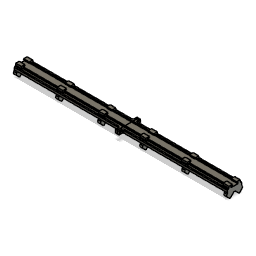
UlTi_LED_Stand (Autodesk Fusion 360 design; units mm, degrees)
Autodesk Fusion 360 part; units mm, degrees
note: some values were not read from the file. Chosen so that the rebuilt part matches the saved one: which bodies a step acts on. Set by a fixed rule: which face or edge a step refers to.
sketch "Sketch1" plane through (0, 0, 0) normal (0, 1, 0) x (1, 0, 0)
  line L0 (0, 0) -> (-300, 0)
  line L1 (-300, 0) -> (-300, 20)
  line L2 (-300, 20) -> (0, 20)
  line L3 (0, 20) -> (0, 0)
  line L4 (-300, 10) -> (0, 10)
  line L5 (-300, 10) -> (-300, 14)
  line L6 (-300, 14) -> (0, 14)
  line L7 (0, 14) -> (0, 6)
  line L8 (0, 6) -> (-300, 6)
  line L9 (-300, 6) -> (-300, 14)
  line L10 (-300, 14) -> (-292, 14)
  line L11 (-292, 14) -> (-292, 18)
  line L12 (-292, 18) -> (-300, 18)
  line L13 (-300, 18) -> (-300, 14)
  line L14 (-300, 16) -> (-292, 16)
  line L15 (-292, 16) -> (-292, 13)
  line L16 (-292, 13) -> (-300, 13)
  line L17 (-300, 13) -> (-300, 16)
  line L18 (-150, 20) -> (-150, 0)
  line L19 (-233.6, 13) -> (-241.6, 13)
  line L20 (-233.6, 16) -> (-233.6, 13)
  line L21 (-241.6, 13) -> (-241.6, 16)
  line L22 (-241.6, 16) -> (-233.6, 16)
  line L23 (-233.6, 18) -> (-241.6, 18)
  line L24 (-233.6, 14) -> (-233.6, 18)
  line L25 (-241.6, 18) -> (-241.6, 14)
  line L26 (-175.2, 13) -> (-183.2, 13)
  line L27 (-175.2, 16) -> (-175.2, 13)
  line L28 (-183.2, 13) -> (-183.2, 16)
  line L29 (-183.2, 16) -> (-175.2, 16)
  line L30 (-175.2, 18) -> (-183.2, 18)
  line L31 (-175.2, 14) -> (-175.2, 18)
  line L32 (-183.2, 18) -> (-183.2, 14)
  line L33 (-116.8, 13) -> (-124.8, 13)
  line L34 (-116.8, 16) -> (-116.8, 13)
  line L35 (-124.8, 13) -> (-124.8, 16)
  line L36 (-124.8, 16) -> (-116.8, 16)
  line L37 (-116.8, 18) -> (-124.8, 18)
  line L38 (-116.8, 14) -> (-116.8, 18)
  line L39 (-124.8, 18) -> (-124.8, 14)
  line L40 (-58.4, 13) -> (-66.4, 13)
  line L41 (-58.4, 16) -> (-58.4, 13)
  line L42 (-66.4, 13) -> (-66.4, 16)
  line L43 (-66.4, 16) -> (-58.4, 16)
  line L44 (-58.4, 18) -> (-66.4, 18)
  line L45 (-58.4, 14) -> (-58.4, 18)
  line L46 (-66.4, 18) -> (-66.4, 14)
  line L47 (0, 13) -> (-8, 13)
  line L48 (0, 16) -> (0, 13)
  line L49 (-8, 13) -> (-8, 16)
  line L50 (-8, 16) -> (0, 16)
  line L51 (0, 18) -> (-8, 18)
  line L52 (0, 14) -> (0, 18)
  line L53 (-8, 18) -> (-8, 14)
  line L54 (-300, 4) -> (-292, 4)
  line L55 (-292, 6) -> (-292, 2)
  line L56 (-292, 2) -> (-300, 2)
  line L57 (-292, 7) -> (-300, 7)
  line L58 (-300, 2) -> (-300, 6)
  line L59 (-300, 20) -> (-300, 0)
  line L60 (-292, 4) -> (-292, 7)
  line L61 (-241.6, 7) -> (-241.6, 4)
  line L62 (-241.6, 4) -> (-233.6, 4)
  line L63 (-241.6, 2) -> (-241.6, 6)
  line L64 (-233.6, 2) -> (-241.6, 2)
  line L65 (-233.6, 7) -> (-241.6, 7)
  line L66 (-300, 6) -> (0, 6)
  line L67 (-233.6, 4) -> (-233.6, 7)
  line L68 (-233.6, 6) -> (-233.6, 2)
  line L69 (-183.2, 2) -> (-183.2, 6)
  line L70 (-175.2, 2) -> (-183.2, 2)
  line L71 (-183.2, 4) -> (-175.2, 4)
  line L72 (-175.2, 7) -> (-183.2, 7)
  line L73 (-183.2, 7) -> (-183.2, 4)
  line L74 (-175.2, 4) -> (-175.2, 7)
  line L75 (-175.2, 6) -> (-175.2, 2)
  line L76 (-124.8, 7) -> (-124.8, 4)
  line L77 (-124.8, 4) -> (-116.8, 4)
  line L78 (-124.8, 2) -> (-124.8, 6)
  line L79 (-116.8, 2) -> (-124.8, 2)
  line L80 (-116.8, 7) -> (-124.8, 7)
  line L81 (-116.8, 4) -> (-116.8, 7)
  line L82 (-116.8, 6) -> (-116.8, 2)
  line L83 (-66.4, 2) -> (-66.4, 6)
  line L84 (-66.4, 4) -> (-58.4, 4)
  line L85 (-58.4, 2) -> (-66.4, 2)
  line L86 (-58.4, 6) -> (-58.4, 2)
  line L87 (-58.4, 7) -> (-66.4, 7)
  line L88 (-58.4, 4) -> (-58.4, 7)
  line L89 (-66.4, 7) -> (-66.4, 4)
  line L90 (-8, 2) -> (-8, 6)
  line L91 (-8, 4) -> (0, 4)
  line L92 (0, 2) -> (-8, 2)
  line L93 (0, 0) -> (0, 20)
  line L94 (0, 7) -> (-8, 7)
  line L95 (-8, 7) -> (-8, 4)
  line L96 (-300, 16) -> (0, 16)
  line L97 (-300, 4) -> (0, 4)
  dimension "d1" = 300
  dimension "d2" = 20
  dimension "d3" = 4
  dimension "d4" = 300
  dimension "d5" = 8
  dimension "d6" = 8
  dimension "d7" = 4
  dimension "d8" = 8
  dimension "d9" = 3
  dimension "d12" = 292
  dimension "d13" = 0
  dimension "d14" = 300
  dimension "d15" = 300
  dimension "d16" = 8
  dimension "d17" = 8
  dimension "d18" = 3
  dimension "d19" = 4
  constraint horizontal L0
  constraint vertical L1
  constraint horizontal L2
  constraint vertical L3
  constraint coincident L0.start L3.end
  constraint midpoint L1 L4.start
  constraint midpoint L3 L4.end
  constraint perpendicular L2 L5
  constraint horizontal L6
  constraint vertical L7
  constraint horizontal L8
  constraint vertical L9
  constraint horizontal L10
  constraint vertical L11
  constraint horizontal L12
  constraint vertical L13
  constraint horizontal L14
  constraint vertical L15
  constraint horizontal L16
  constraint vertical L17
  constraint midpoint L13 L14.start
  constraint midpoint L2 L18.start
  constraint midpoint L0 L18.end
  constraint symmetric L0.start L4 L2.end
  constraint symmetric L0.end L4 L1.end
  constraint symmetric L1.end L4 L0.end
  constraint symmetric L2.end L4 L0.start
  constraint symmetric L4 L5.end L8.end
  constraint symmetric L4 L6.end L7.end
  constraint symmetric L4 L10.end L55.start
  constraint symmetric L4 L11.end L55.end
  constraint symmetric L4 L12.end L56.end
  constraint symmetric L4 L14.start L54.start
  constraint symmetric L4 L14.end L54.end
  constraint symmetric L4 L15.end L57.start
  constraint symmetric L4 L16.end L57.end
  constraint symmetric L4 L19.start L65.start
  constraint symmetric L4 L19.end L61.start
  constraint symmetric L4 L20.start L62.end
  constraint symmetric L4 L21.end L61.end
  constraint symmetric L4 L23.start L64.start
  constraint symmetric L4 L23.end L63.start
  constraint symmetric L4 L24.start L68.start
  constraint symmetric L4 L25.end L63.end
  constraint symmetric L4 L26.start L72.start
  constraint symmetric L4 L26.end L72.end
  constraint symmetric L4 L27.start L71.end
  constraint symmetric L4 L28.end L71.start
  constraint symmetric L4 L30.start L70.start
  constraint symmetric L4 L30.end L69.start
  constraint symmetric L4 L31.start L75.start
  constraint symmetric L4 L32.end L69.end
  constraint symmetric L4 L33.start L80.start
  constraint symmetric L4 L33.end L76.start
  constraint symmetric L4 L34.start L77.end
  constraint symmetric L4 L35.end L76.end
  constraint symmetric L4 L37.start L79.start
  constraint symmetric L4 L37.end L78.start
  constraint symmetric L4 L38.start L82.start
  constraint symmetric L4 L39.end L78.end
  constraint symmetric L4 L40.start L87.start
  constraint symmetric L4 L40.end L87.end
  constraint symmetric L4 L41.start L84.end
  constraint symmetric L4 L42.end L84.start
  constraint symmetric L4 L44.start L85.start
  constraint symmetric L4 L44.end L83.start
  constraint symmetric L4 L45.start L86.start
  constraint symmetric L4 L46.end L83.end
  constraint symmetric L4 L47.start L94.start
  constraint symmetric L4 L47.end L94.end
  constraint symmetric L4 L48.start L91.end
  constraint symmetric L4 L49.end L91.start
  constraint symmetric L4 L51.start L92.start
  constraint symmetric L4 L51.end L90.start
  constraint symmetric L4 L53.end L90.end
  constraint horizontal L96
  measures "d1" distance of L0.start L0.end
  measures "d2" distance of L0.start L2.end
  measures "d3" distance of L4.start L5.end
  measures "d4" distance of L5.end L6.end
  measures "d5" distance of L5.end L8.end
  measures "d6" distance of L5.end L10.end
  measures "d7" distance of L5.end L12.end
  measures "d8" distance of L14.start L14.end
  measures "d9" distance of L14.start L16.end
  measures "d14" distance of L14.start L48.start
  measures "d15" distance of L1.end L2.end
  measures "d16" distance of L55.end L56.end
  measures "d17" distance of L57.start L57.end
  measures "d18" distance of L54.end L57.start
  measures "d19" distance of L55.start L55.end
extrude "Extrude1" add sketch "Sketch1" along normal blind 5 makes body 1
extrude "Extrude2" add sketch "Sketch1" along normal blind 6 contours L8 L18 L66 L74 L75 L97 | L8 L18 L66 L76 L78 L97 | L3 L8 L66 L90 L91 L93 L95 L97 | L8 L66 L69 L71 L73 L74 L75 L97 | L8 L66 L76 L77 L78 L81 L82 L97 | L8 L66 L86 L88 L90 L95 L97 | L1 L8 L54 L55 L58 L59 L60 L66 L97 | L8 L66 L67 L68 L69 L73 L97 | L8 L66 L81 L82 L83 L89 L97 | L8 L66 L83 L84 L86 L88 L89 L97 | L8 L55 L60 L61 L63 L66 L97 | L6 L18 L35 L39 L96 | L6 L18 L27 L31 L96 | L8 L61 L62 L63 L66 L67 L68 L97 | L6 L27 L28 L29 L31 L32 L96 | L6 L34 L35 L36 L38 L39 L96 | L1 L6 L10 L11 L13 L14 L15 L17 L59 L96 | L3 L6 L48 L49 L50 L52 L53 L93 L96 | L6 L20 L24 L28 L32 L96 | L6 L34 L38 L42 L46 L96 | L6 L11 L15 L21 L25 L96 | L6 L41 L45 L49 L53 L96 | L6 L20 L21 L22 L24 L25 L96 | L6 L41 L42 L43 L45 L46 L96 bodies 1
extrude "Extrude3" add sketch "Sketch1" along normal blind 7 contours L3 L90 L91 L92 L93 L97 | L3 L8 L66 L90 L91 L93 L95 L97 | L1 L54 L55 L56 L58 L59 L97 | L69 L70 L71 L75 L97 | L8 L66 L69 L71 L73 L74 L75 L97 | L8 L66 L76 L77 L78 L81 L82 L97 | L77 L78 L79 L82 L97 | L3 L7 L8 L66 L93 L94 L95 | L1 L8 L54 L55 L58 L59 L60 L66 L97 | L8 L66 L76 L80 L81 | L8 L66 L72 L73 L74 | L83 L84 L85 L86 L97 | L8 L66 L83 L84 L86 L88 L89 L97 | L1 L8 L9 L57 L59 L60 L66 | L62 L63 L64 L68 L97 | L8 L61 L62 L63 L66 L67 L68 L97 | L8 L66 L87 L88 L89 | L8 L61 L65 L66 L67 | L1 L5 L6 L9 L10 L15 L16 L17 L59 | L3 L6 L7 L47 L48 L49 L93 | L6 L26 L27 L28 | L6 L27 L28 L29 L31 L32 L96 | L6 L34 L35 L36 L38 L39 L96 | L6 L33 L34 L35 | L1 L6 L10 L11 L13 L14 L15 L17 L59 L96 | L3 L6 L48 L49 L50 L52 L53 L93 L96 | L29 L30 L31 L32 L96 | L36 L37 L38 L39 L96 | L1 L11 L12 L13 L14 L59 L96 | L3 L50 L51 L52 L53 L93 L96 | L6 L19 L20 L21 | L6 L20 L21 L22 L24 L25 L96 | L6 L41 L42 L43 L45 L46 L96 | L6 L40 L41 L42 | L22 L23 L24 L25 L96 | L43 L44 L45 L46 L96 bodies 1
ref_plane "WorkPlane1" through (-62.4, 6, -4.5) normal (0, 1, 0) x (0, 0, 1)
sketch "Sketch2" plane through (0, 6, 0) normal (0, 1, 0) x (1, 0, 0)
  line L0 (0, 2) -> (0, 7)
  line L1 (0, 7) -> (-8, 7)
  line L2 (-8, 7) -> (-8, 2)
  line L3 (-8, 2) -> (0, 2)
  line L4 (0, 13) -> (0, 18)
  line L5 (0, 18) -> (-8, 18)
  line L6 (-8, 18) -> (-8, 13)
  line L7 (-8, 13) -> (0, 13)
  line L8 (-58.4, 2) -> (-58.4, 7)
  line L9 (-58.4, 7) -> (-66.4, 7)
  line L10 (-66.4, 7) -> (-66.4, 2)
  line L11 (-66.4, 2) -> (-58.4, 2)
  line L12 (-58.4, 13) -> (-58.4, 18)
  line L13 (-58.4, 18) -> (-66.4, 18)
  line L14 (-66.4, 18) -> (-66.4, 13)
  line L15 (-66.4, 13) -> (-58.4, 13)
  line L16 (-116.8, 13) -> (-116.8, 18)
  line L17 (-116.8, 18) -> (-124.8, 18)
  line L18 (-124.8, 18) -> (-124.8, 13)
  line L19 (-124.8, 13) -> (-116.8, 13)
  line L20 (-116.8, 7) -> (-124.8, 7)
  line L21 (-124.8, 7) -> (-124.8, 2)
  line L22 (-124.8, 2) -> (-116.8, 2)
  line L23 (-116.8, 2) -> (-116.8, 7)
  line L24 (-175.2, 7) -> (-183.2, 7)
  line L25 (-183.2, 7) -> (-183.2, 2)
  line L26 (-183.2, 2) -> (-175.2, 2)
  line L27 (-175.2, 2) -> (-175.2, 7)
  line L28 (-175.2, 13) -> (-175.2, 18)
  line L29 (-175.2, 18) -> (-183.2, 18)
  line L30 (-183.2, 18) -> (-183.2, 13)
  line L31 (-183.2, 13) -> (-175.2, 13)
  line L32 (-233.6, 13) -> (-233.6, 18)
  line L33 (-233.6, 18) -> (-241.6, 18)
  line L34 (-241.6, 18) -> (-241.6, 13)
  line L35 (-241.6, 13) -> (-233.6, 13)
  line L36 (-233.6, 7) -> (-241.6, 7)
  line L37 (-241.6, 7) -> (-241.6, 2)
  line L38 (-241.6, 2) -> (-233.6, 2)
  line L39 (-233.6, 2) -> (-233.6, 7)
  line L40 (-292, 13) -> (-292, 18)
  line L41 (-292, 18) -> (-300, 18)
  line L42 (-300, 18) -> (-300, 13)
  line L43 (-300, 13) -> (-292, 13)
  line L44 (-292, 2) -> (-292, 7)
  line L45 (-292, 7) -> (-300, 7)
  line L46 (-300, 7) -> (-300, 2)
  line L47 (-300, 2) -> (-292, 2)
  line L48 (-292, 7) -> (-300, 7)
  line L49 (-300, 7) -> (-300, 6)
  line L50 (-300, 6) -> (-292, 6)
  line L51 (-292, 6) -> (-292, 7)
  line L52 (-241.6, 6) -> (-233.6, 6)
  line L53 (-233.6, 6) -> (-233.6, 7)
  line L54 (-233.6, 7) -> (-241.6, 7)
  line L55 (-241.6, 7) -> (-241.6, 6)
  line L56 (-183.2, 6) -> (-175.2, 6)
  line L57 (-175.2, 6) -> (-175.2, 7)
  line L58 (-175.2, 7) -> (-183.2, 7)
  line L59 (-183.2, 7) -> (-183.2, 6)
  line L60 (-124.8, 6) -> (-116.8, 6)
  line L61 (-116.8, 6) -> (-116.8, 7)
  line L62 (-116.8, 7) -> (-124.8, 7)
  line L63 (-124.8, 7) -> (-124.8, 6)
  line L64 (-66.4, 6) -> (-58.4, 6)
  line L65 (-58.4, 6) -> (-58.4, 7)
  line L66 (-58.4, 7) -> (-66.4, 7)
  line L67 (-66.4, 7) -> (-66.4, 6)
  line L68 (-8, 6) -> (0, 6)
  line L69 (0, 6) -> (0, 7)
  line L70 (0, 7) -> (-8, 7)
  line L71 (-8, 7) -> (-8, 6)
  line L72 (0, 0) -> (0, 10)
  line L73 (0, 10) -> (-300, 10)
  line L74 (0, 10) -> (-300, 10)
  line L75 (-8, 14) -> (0, 14)
  line L76 (0, 14) -> (0, 13)
  line L77 (0, 13) -> (-8, 13)
  line L78 (-8, 13) -> (-8, 14)
  line L79 (-58.4, 13) -> (-66.4, 13)
  line L80 (-58.4, 13) -> (-66.4, 13)
  line L81 (-58.4, 14) -> (-58.4, 13)
  line L82 (-66.4, 14) -> (-58.4, 14)
  line L83 (-66.4, 13) -> (-66.4, 14)
  line L84 (-116.8, 14) -> (-116.8, 13)
  line L85 (-124.8, 14) -> (-116.8, 14)
  line L86 (-116.8, 13) -> (-124.8, 13)
  line L87 (-116.8, 13) -> (-124.8, 13)
  line L88 (-124.8, 13) -> (-124.8, 14)
  line L89 (-183.2, 13) -> (-183.2, 14)
  line L90 (-175.2, 13) -> (-183.2, 13)
  line L91 (-175.2, 13) -> (-183.2, 13)
  line L92 (-183.2, 14) -> (-175.2, 14)
  line L93 (-175.2, 14) -> (-175.2, 13)
  line L94 (-241.6, 13) -> (-241.6, 14)
  line L95 (-241.6, 14) -> (-233.6, 14)
  line L96 (-233.6, 13) -> (-241.6, 13)
  line L97 (-233.6, 14) -> (-233.6, 13)
  line L98 (-233.6, 13) -> (-241.6, 13)
  line L99 (-300, 13) -> (-300, 14)
  line L100 (-292, 13) -> (-300, 13)
  line L101 (-300, 14) -> (-292, 14)
  line L102 (-292, 13) -> (-300, 13)
  line L103 (-292, 14) -> (-292, 13)
  dimension "d27" = 1
  dimension "d30" = 292
  dimension "d31" = 0
  dimension "d32" = 10
  dimension "d33" = 90
  dimension "d34" = 300
  constraint horizontal L48
  constraint vertical L49
  constraint horizontal L50
  constraint vertical L51
  constraint coincident L44.end L45.start
  constraint coincident L72.start origin
  constraint perpendicular L1 L72
  constraint symmetric L8.end L73 L12.start
  constraint symmetric L9.end L73 L14.end
  constraint symmetric L20.start L73 L16.start
  constraint symmetric L20.end L73 L18.end
  constraint symmetric L24.start L73 L28.start
  constraint symmetric L24.end L73 L30.end
  constraint symmetric L36.start L73 L32.start
  constraint symmetric L36.end L73 L34.end
  constraint symmetric L44.end L73 L40.start
  constraint symmetric L45.end L73 L42.end
  constraint symmetric L49.end L73 L99.end
  constraint symmetric L50.end L73 L101.end
  constraint symmetric L52.start L73 L94.end
  constraint symmetric L52.end L73 L95.end
  constraint symmetric L56.start L73 L89.end
  constraint symmetric L56.end L73 L92.end
  constraint symmetric L60.start L73 L85.start
  constraint symmetric L60.end L73 L84.start
  constraint symmetric L64.start L73 L82.start
  constraint symmetric L64.end L73 L81.start
  constraint symmetric L68.start L73 L75.start
  constraint symmetric L68.end L73 L75.end
  constraint symmetric L0.end L73 L4.start
  constraint symmetric L1.end L73 L6.end
  constraint symmetric L72.end L73 L74.start
  constraint symmetric L74.end L73 L73.end
  measures "d27" distance of L44.end L50.end
  measures "d32" distance of L72.start L72.end
  measures "d33" angle of L72 L73
  measures "d34" distance of L72.end L73.end
extrude "Extrude4" cut sketch "Sketch2" against normal blind 1 contours L0 L1 L2 L68 L69 L70 L71 L72 | L4 L6 L7 L75 L76 L77 L78 | L8 L9 L10 L64 L65 L66 L67 | L12 L14 L15 L79 L80 L81 L82 L83 | L16 L18 L19 L84 L85 L86 L87 L88 | L20 L21 L23 L60 L61 L62 L63 | L24 L25 L27 L56 L57 L58 L59 | L28 L30 L31 L89 L90 L91 L92 L93 | L32 L34 L35 L94 L95 L96 L97 L98 | L36 L37 L39 L52 L53 L54 L55 | L40 L42 L43 L99 L100 L101 L102 L103 | L44 L45 L46 L48 L49 L50 L51 bodies 1
sketch "Sketch3" plane through (-300, 0, 0) normal (-1, 0, 0) x (0, 0, 1)
  line L0 (-7, 6) -> (-6, 6)
  line L1 (-6, 6) -> (-6, 5)
  line L2 (-6, 5) -> (-14, 5)
  line L3 (-14, 5) -> (-14, 6)
  line L4 (-14, 6) -> (-13, 6)
  line L5 (-13, 6) -> (-13, 7)
  line L6 (-13, 7) -> (-18, 7)
  line L7 (-18, 7) -> (-18, 5)
  line L8 (-18, 5) -> (-20, 5)
  line L9 (-20, 5) -> (-20, 0)
  line L10 (-20, 0) -> (0, 0)
  line L11 (0, 0) -> (0, 5)
  line L12 (0, 5) -> (-2, 5)
  line L13 (-2, 5) -> (-2, 7)
  line L14 (-2, 7) -> (-7, 7)
  line L15 (-7, 7) -> (-7, 6)
  line L16 (-10, 0) -> (-10, -18.1592)
  line L17 (-20, 0) -> (-10, -10)
  line L18 (-20, 0) -> (-5.8579, 0) construction
  line L19 (-10, -10) -> (0, 0)
  line L20 (-18.2322, 1.7678) -> (-10, -6.4645)
  line L21 (-10, -6.4645) -> (-1.7678, 1.7678)
  line L22 (-10, 0) -> (-11, 0)
  line L23 (-11, 0) -> (-11, -6.4645)
  line L24 (-11, -6.4645) -> (-10, -6.4645)
  line L25 (-10, -6.4645) -> (-10, 0)
  line L26 (-9, 0) -> (-9, -6.4645)
  line L27 (-9, -6.4645) -> (-10, -6.4645)
  line L28 (-11, 0) -> (-11, -2.2)
  line L29 (-11, -2.2) -> (-14.4, -5.6)
  line L30 (-11, -2.2) -> (-9, -2.2)
  line L31 (-9, -2.2) -> (-5.6, -5.6)
  line L32 (-9, -2.2) -> (-11, -2.2)
  dimension "d37" = 45
  dimension "d38" = -2.5
  dimension "d39" = 1
  dimension "d40" = 1
  dimension "d52" = 2.2
  dimension "d53" = 7.8
  constraint midpoint L10 L16.start
  constraint perpendicular L10 L16
  constraint horizontal L18
  constraint coincident L9.end L10.start
  constraint coincident L16 L17.end
  constraint coincident L10.end L11.start
  constraint perpendicular L22 L23
  constraint parallel L22 L24
  constraint parallel L23 L25
  constraint perpendicular L16 L22
  constraint symmetric L16 L22.end L26.start
  constraint symmetric L16 L23.end L26.end
  constraint perpendicular L25 L27
  constraint perpendicular L18 L28
  constraint coincident L17 L29.end
  constraint perpendicular L17 L29
  constraint coincident L26 L30.end
  constraint perpendicular L26 L30
  constraint symmetric L25 L28.end L30.end
  constraint symmetric L25 L29.end L31.end
  constraint symmetric L25 L30.end L28.end
  measures "d37" angle of L17 L18
  measures "d39" distance of L16.start L22.end
  measures "d40" distance of L20.end L23.end
  measures "d52" distance of L22.end L28.end
  measures "d53" vertical distance of L17.end L30.end
sketch "Sketch4" plane through (0, 0, 0) normal (0, 0, 1) x (1, 0, 0)
  line L0 (-300, 0) -> (0, 0)
  line L1 (0, 0) -> (0, 5)
  line L2 (0, 5) -> (-300, 5)
  line L3 (-300, 5) -> (-300, 0)
  line L4 (0, 0) -> (-150, 0)
  line L5 (-150, 0) -> (-150, 2.5)
  line L6 (-153, 5) -> (-147, 5)
  line L7 (-147, 5) -> (-147, 0)
  line L8 (-147, 0) -> (-153, 0)
  line L9 (-153, 0) -> (-153, 5)
  line L10 (-153, 5) -> (-147, 0) construction
  line L11 (-147, 5) -> (-153, 0) construction
  point P0 (-150, 2.5)
  dimension "d41" = 150
  dimension "d42" = 2.5
  dimension "d43" = 6
  dimension "d44" = 5
  constraint coincident L0.end L1.start
  constraint perpendicular L1 L4
  constraint perpendicular L4 L5
  constraint horizontal L6
  constraint perpendicular L6 L7
  constraint parallel L6 L8
  constraint parallel L7 L9
  constraint coincident L10 P0
  constraint coincident L11 P0
  constraint coincident P0 L5.end
  measures "d41" distance of L0.end L4.end
  measures "d42" distance of L4.end P0
  measures "d43" distance of L7.end L8.end
  measures "d44" distance of L6.end L7.end
extrude "Extrude5" add sketch "Sketch4" along normal blind 5 contours L0 L2 L4 L6 L7 L8 L9 bodies 1
sketch "Sketch5" plane through (-147, 0, 0) normal (1, 0, 0) x (0, 0, -1)
  line L0 (0, 0) -> (0, 5)
  line L1 (0, 5) -> (-5, 5)
  line L2 (-5, 5) -> (-5, 0)
  line L3 (-5, 0) -> (0, 0)
  line L4 (-5, 5) -> (-2.5, 2.5)
  circle A0 centre (-2.5, 2.5) radius 1.5
  line L5 (0, 5) -> (10, 5)
  line L6 (10, 5) -> (10, 0)
  line L7 (20, 5) -> (25, 5)
  circle A1 centre (22.5, 2.5) radius 1.5
  line L8 (20, 0) -> (20, 5)
  line L9 (25, 0) -> (20, 0)
  line L10 (25, 5) -> (22.5, 2.5)
  line L11 (25, 5) -> (25, 0)
  point P0 (20, 0)
  point P1 (20, 5)
  dimension "d47" = 3
  dimension "d48" = 10
  dimension "d49" = 5
  constraint coincident L1.end L2.start
  constraint coincident L4.end A0.centre
  constraint coincident L0.end L1.start
  constraint perpendicular L0 L5
  constraint perpendicular L5 L6
  constraint symmetric L0.start L6 L8.start
  constraint symmetric L0.start L6 P0
  constraint symmetric L0.end L6 P1
  constraint symmetric L1.end L6 L7.end
  constraint symmetric L2.end L6 L9.start
  constraint symmetric L4.end L6 A1.centre
  constraint symmetric A0 L6 A1
  measures "d47" diameter of A0
  measures "d48" distance of L0.end L5.end
  measures "d49" distance of L5.end L6.end
extrude "Extrude6" add sketch "Sketch5" against normal blind 6 contours L7 L8 L9 L11 bodies 1
extrude "Extrude7" add sketch "Sketch3" against normal blind 4 contours L10 L19 L21 L31 | L10 L21 L26 L31 | L10 L16 L25 L26 L30 L32 | L10 L16 L22 L23 L25 L28 L30 L32 | L10 L17 L20 L29 | L10 L20 L23 L28 L29 bodies 1
ref_plane "WorkPlane2" through (-148, 0, -10) normal (0, -1, 0) x (-1, 0, 0)
split "Split1" by plane through (-148, 0, -10) normal (0, -1, 0) bodies 1 makes body 2 at (-296, -2.6, -15.1333)
pattern_linear "R-Pattern1" count 6 spacing 59.2 along (1, 0, 0) of bodies 2 makes body 3 at (-239.4667, 0, -6.6667) makes body 4 at (-180.2667, 0, -6.6667) makes body 5 at (-121.0667, 0, -6.6667) makes body 6 at (-61.8667, 0, -6.6667) makes body 7 at (-2.6667, 0, -6.6667)
combine "Combine1" operation add target body 1 tool bodies 3 2 4 5 6 7
fillet "Fillet1" radius 1 4 edges at (-153, 2.5, -20) (-147, 2.5, -20) (-147, 2.5, 0) (-153, 2.5, 0) on bodies 1
extrude "Extrude8" cut sketch "Sketch5" against normal blind 21 contours A0 bodies 1
fillet "Fillet2" radius 1 16 edges at (-147, 5, 3) (-146.7071, 5, 0.2929) (-73, 5, 0) (-134.2, 0, 0) (-146.7071, 0, 0.2929) (-147, 0, 3) (-90.8, 0, 0) (-31.6, 0, 0) (-73, 5, -20) (-146.7071, 5, -20.2929) (-147, 5, -23) (-31.6, 0, -20) (-90.8, 0, -20) (-147, 0, -23) (-146.7071, 0, -20.2929) (-134.2, 0, -20) on bodies 1
fillet "Fillet3" radius 1 16 edges at (-153, 5, -23) (-153.2929, 5, -20.2929) (-227, 5, -20) (-209.2, 0, -20) (-165.8, 0, -20) (-153.2929, 0, -20.2929) (-153, 0, -23) (-268.4, 0, -20) (-227, 5, 0) (-153.2929, 5, 0.2929) (-153, 5, 3) (-268.4, 0, 0) (-209.2, 0, 0) (-153, 0, 3) (-153.2929, 0, 0.2929) (-165.8, 0, 0) on bodies 1
fillet "Fillet4" radius 0.25 8 edges at (-152.7071, 0.2929, 5) (-150, 0, 5) (-147.2929, 0.2929, 5) (-147, 2.5, 5) (-147.2929, 4.7071, 5) (-150, 5, 5) (-152.7071, 4.7071, 5) (-153, 2.5, 5) on bodies 1
fillet "Fillet5" radius 0.5 8 edges at (-150, 0, -25) (-147.2929, 0.2929, -25) (-147, 2.5, -25) (-147.2929, 4.7071, -25) (-150, 5, -25) (-152.7071, 4.7071, -25) (-153, 2.5, -25) (-152.7071, 0.2929, -25) on bodies 1
fillet "Fillet6" radius 0.5 42 edges at (-266.8, 5, -16) (-241.6, 5, -17) (-237.6, 5, -18) (-296, 5, -18) (-292, 5, -17) (-233.6, 5, -17) (-208.4, 5, -16) (-179.2, 5, -18) (-150, 5, -16) (-175.2, 5, -17) (-183.2, 5, -17) (-120.8, 5, -18) (-124.8, 5, -17) (-91.6, 5, -16) (-116.8, 5, -17) (-62.4, 5, -18) (-58.4, 5, -17) (-33.2, 5, -16) (-66.4, 5, -17) (-4, 5, -18) (-8, 5, -17) (-33.2, 5, -4) (-8, 5, -3) (-4, 5, -2) (-62.4, 5, -2) (-66.4, 5, -3) (-91.6, 5, -4) (-58.4, 5, -3) (-116.8, 5, -3) (-120.8, 5, -2) (-150, 5, -4) (-124.8, 5, -3) (-179.2, 5, -2) (-183.2, 5, -3) (-208.4, 5, -4) (-175.2, 5, -3) (-233.6, 5, -3) (-237.6, 5, -2) (-241.6, 5, -3) (-266.8, 5, -4) (-296, 5, -2) (-292, 5, -3) on bodies 1
sketch "Sketch6" plane through (-300, 0, 0) normal (-1, 0, 0) x (0, 0, 1)
  arc A0 (0, 4) -> (-1, 5) centre (-1, 4) ccw
  line L0 (-1, 5) -> (-1.5, 5)
  arc A1 (-2, 5.5) -> (-1.5, 5) centre (-1.5, 5.5) ccw
  line L1 (-2, 5.5) -> (-2, 7)
  line L2 (-2, 7) -> (-7, 7)
  line L3 (-7, 7) -> (-7, 6)
  line L4 (-7, 6) -> (-6, 6)
  line L5 (-6, 6) -> (-6, 5)
  line L6 (-6, 5) -> (-14, 5)
  line L7 (-14, 5) -> (-14, 6)
  line L8 (-14, 6) -> (-13, 6)
  line L9 (-13, 6) -> (-13, 7)
  line L10 (-13, 7) -> (-18, 7)
  line L11 (-18, 7) -> (-18, 5.5)
  arc A2 (-18.5, 5) -> (-18, 5.5) centre (-18.5, 5.5) ccw
  line L12 (-18.5, 5) -> (-19, 5)
  arc A3 (-19, 5) -> (-20, 4) centre (-19, 4) ccw
  line L13 (-20, 4) -> (-20, 0)
  line L14 (-20, 0) -> (-14.4, -5.6)
  line L15 (-14.4, -5.6) -> (-11, -2.2)
  line L16 (-11, -2.2) -> (-9, -2.2)
  line L17 (-9, -2.2) -> (-5.6, -5.6)
  line L18 (-5.6, -5.6) -> (0, 0)
  line L19 (0, 0) -> (0, 4)
  line L20 (-14, 6) -> (-15, 6)
  line L21 (-15, 6) -> (-15, 5)
  line L22 (-15, 5) -> (-14, 5)
  line L23 (-14, 5) -> (-14, 6)
  line L24 (-6, 6) -> (-5, 6)
  line L25 (-5, 6) -> (-5, 5)
  line L26 (-5, 5) -> (-6, 5)
  line L27 (-6, 5) -> (-6, 6)
  line L28 (-14, 6) -> (-13, 6)
  line L29 (-13, 6) -> (-13, 6.4)
  line L30 (-13, 6.4) -> (-14, 6.4)
  line L31 (-14, 6.4) -> (-14, 6)
  line L32 (-6, 6) -> (-7, 6)
  line L33 (-7, 6) -> (-7, 6.4)
  line L34 (-7, 6.4) -> (-6, 6.4)
  line L35 (-6, 6.4) -> (-6, 6)
  line L36 (-18, 7) -> (-13, 7)
  line L37 (-13, 7) -> (-13, 8)
  line L38 (-13, 8) -> (-18, 8)
  line L39 (-18, 8) -> (-18, 7)
  line L40 (-7, 7) -> (-2, 7)
  line L41 (-2, 7) -> (-2, 8)
  line L42 (-2, 8) -> (-7, 8)
  line L43 (-7, 8) -> (-7, 7)
  line L44 (-14, 6) -> (-15, 6)
  line L45 (-15, 6) -> (-15, 6.4)
  line L46 (-15, 6.4) -> (-14, 6.4)
  line L47 (-14, 6.4) -> (-14, 6)
  line L48 (-6, 6) -> (-5, 6)
  line L49 (-5, 6) -> (-5, 6.4)
  line L50 (-5, 6.4) -> (-6, 6.4)
  line L51 (-6, 6.4) -> (-6, 6)
  dimension "d75" = 1
  dimension "d76" = 1
  dimension "d77" = 1
  dimension "d78" = 1
  dimension "d79" = 0.4
  dimension "d80" = 1
  dimension "d81" = 0.4
  dimension "d82" = 5
  dimension "d83" = 1
  dimension "d84" = 5
  dimension "d85" = 1
  dimension "d90" = 4
  dimension "d91" = 0.4
  dimension "d92" = 1
  dimension "d93" = 0.4
  constraint horizontal L20
  constraint vertical L21
  constraint horizontal L22
  constraint vertical L23
  constraint coincident L7.end L8.start
  constraint horizontal L24
  constraint vertical L25
  constraint horizontal L26
  constraint vertical L27
  constraint coincident L4.end L5.start
  constraint horizontal L28
  constraint vertical L29
  constraint horizontal L30
  constraint vertical L31
  constraint coincident L9 L29.end
  constraint horizontal L32
  constraint vertical L33
  constraint horizontal L34
  constraint vertical L35
  constraint horizontal L36
  constraint vertical L37
  constraint horizontal L38
  constraint vertical L39
  constraint coincident L10.end L11.start
  constraint horizontal L40
  constraint vertical L41
  constraint horizontal L42
  constraint vertical L43
  constraint coincident L2.end L3.start
  constraint horizontal L44
  constraint vertical L45
  constraint horizontal L46
  constraint vertical L47
  constraint horizontal L48
  constraint vertical L49
  constraint horizontal L50
  constraint vertical L51
  measures "d75" distance of L7.end L20.end
  measures "d76" distance of L7.end L6.end
  measures "d77" distance of L4.end L24.end
  measures "d78" distance of L4.end L5.end
  measures "d79" distance of L7.end L30.end
  measures "d80" distance of L4.end L3.end
  measures "d81" distance of L4.end L34.end
  measures "d82" distance of L10.end L9.end
  measures "d83" distance of L10.end L38.end
  measures "d84" distance of L2.end L1.end
  measures "d85" distance of L2.end L42.end
  measures "d90" distance of L11 L31
  measures "d91" distance of L7.end L30.end
  measures "d92" distance of L4.end L24.end
  measures "d93" distance of L4.end L34.end
extrude "Extrude9" cut sketch "Sketch6" against normal blind 400 contours L8 L9 L28 L29 L30 L31 L47 bodies 1
extrude "Extrude10" cut sketch "Sketch6" against normal blind 400 contours L3 L4 L32 L33 L34 L35 L51 bodies 1
extrude "Extrude11" cut sketch "Sketch6" against normal blind 400 contours L24 L35 L48 L49 L50 L51 | L5 L24 L25 L26 L27 L48 | L7 L20 L21 L22 L23 L44 | L20 L31 L44 L45 L46 L47 bodies 1
extrude "Extrude12" add sketch "Sketch6" against normal blind 8 separate body contours L2 L40 L41 L42 L43 | L10 L36 L37 L38 L39 makes body 8 at (-297.3333, 8, -14.6667) makes body 9 at (-297.3333, 7, -3.6667)
pattern_linear "R-Pattern2" count 6 spacing 58.4 along (1, 0, 0) of bodies 9 8 makes body 10 at (-238.9333, 8, -14.6667) makes body 11 at (-180.5333, 8, -14.6667) makes body 12 at (-122.1333, 8, -14.6667) makes body 13 at (-63.7333, 8, -14.6667) makes body 14 at (-2.6667, 8, -14.6667) makes body 15 at (-238.9333, 7, -3.6667) makes body 16 at (-180.5333, 7, -3.6667) makes body 17 at (-122.1333, 7, -3.6667) makes body 18 at (-63.7333, 7, -3.6667) makes body 19 at (-5.3333, 7, -3.6667)
combine "Combine2" operation add target body 17 tool bodies 11 1 13 19 12 15 18 14 16 8 9 10
extrude "Extrude13" add 6 faces at (-298.6667, -1.8667, -18.1333) (-180.2667, -1.8667, -18.1333) (-239.4667, -1.8667, -18.1333) (-2.6667, -1.8667, -18.1333) (-121.0667, -1.8667, -18.1333) (-61.8667, -1.8667, -18.1333) along direction (0, -0.707107, -0.707107) blind 3 on bodies 17 bodies 17
extrude "Extrude14" add 6 faces at (-239.4667, -3.7333, -3.7333) (-298.6667, -3.7333, -3.7333) (-180.2667, -3.7333, -3.7333) (-2.6667, -1.8667, -1.8667) (-121.0667, -3.7333, -3.7333) (-61.8667, -3.7333, -3.7333) along direction (0, -0.707107, 0.707107) blind 3 on bodies 17 bodies 17
fillet "Fillet7" radius 2.5 24 edges at (-2, 0, 0) (-2, -2.1213, 2.1213) (-61.2, -2.1213, 2.1213) (-61.2, 0, 0) (-120.4, -2.1213, 2.1213) (-120.4, 0, 0) (-179.6, 0, 0) (-179.6, -2.1213, 2.1213) (-238.8, 0, 0) (-238.8, -2.1213, 2.1213) (-298, 0, 0) (-298, -2.1213, 2.1213) (-298, 0, -20) (-298, -2.1213, -22.1213) (-238.8, -2.1213, -22.1213) (-238.8, 0, -20) (-179.6, -2.1213, -22.1213) (-179.6, 0, -20) (-120.4, -2.1213, -22.1213) (-120.4, 0, -20) (-61.2, -2.1213, -22.1213) (-61.2, 0, -20) (-2, -2.1213, -22.1213) (-2, 0, -20) on bodies 17
ref_plane "WorkPlane3" through (-150, 0.1393, -10) normal (1, 0, 0) x (0, 0, -1)
split "Split2" by plane through (-150, 0.1393, -10) normal (1, 0, 0) bodies 17 makes body 20 at (-50, 5, -11.6667)
